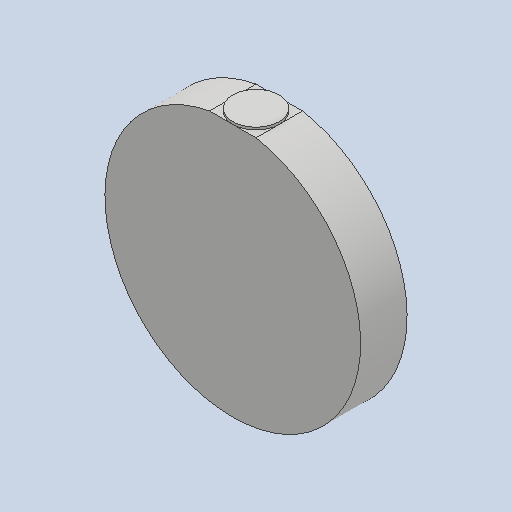
# Autodesk Inventor part: ч ASY human dummy 01
Saved by Autodesk Inventor 2024.2 (Build 282272000, 272)
## iProperties
Created: 2018-05-21
Part Number: ч ASY human dummy 01
Material: Типовые
Document SubType Name: Modeling
Designer: admin
Density: 1 g/cm^3
Appearance: По умолчанию
Author: admin
Autodesk Inventor part; units mm, degrees
ref_plane "YZ Plane" through (0, 0, 0) normal (1, 0, 0) x (0, 1, 0)
ref_plane "XZ Plane" through (0, 0, 0) normal (0, 1, 0) x (-1, 0, 0)
ref_plane "XY Plane" through (0, 0, 0) normal (0, 0, 1) x (1, 0, 0)
sketch "Эскиз1" plane through (0, 0, 0) normal (0, 0, 1) x (1, 0, 0)
  circle A0 centre (0, 0) radius 10
  dimension "d8" = 20
  constraints: 1 centre point, 1 coincident
  measures "d8" diameter of A0
extrude "Выдавливание1" add sketch "Эскиз1" along normal blind 1
sketch "Эскиз3" plane through (0, 0, 0) normal (0, 1, 0) x (-1, 0, 0)
  line L0 (-10, 0) -> (10, 0) projected
  line L1 (-10, 0) -> (10, 0)
  arc A0 (-10, 0) -> (10, 0) centre (0, -54.0833) ccw
  point P0 (0, 0)
  dimension "d5" = 55
  constraints: 2 end point, 2 point on circle, 1 centre point, 1 collinear
  measures "d5" radius of A0
extrude "Выдавливание2" add sketch "Эскиз3" along normal mid plane 20
